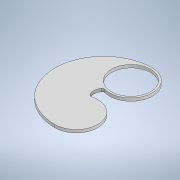
# Autodesk Inventor part: Holder
Saved by Autodesk Inventor 2020 (Build 240168000, 168)
## iProperties
Created: 2020-12-15
Part Number: Holder
Material: Generic
Document SubType Name: Modeling
Designer: moham
Density: 1 g/cm^3
Appearance: Default
Author: moham
Autodesk Inventor part; units mm, degrees
ref_plane "YZ Plane" through (0, 0, 0) normal (1, 0, 0) x (0, 1, 0)
ref_plane "XZ Plane" through (0, 0, 0) normal (0, 1, 0) x (-1, 0, 0)
ref_plane "XY Plane" through (0, 0, 0) normal (0, 0, 1) x (1, 0, 0)
sketch "Sketch1" plane through (0, 0, 0) normal (0, 1, 0) x (-1, 0, 0)
  arc A0 (0, -50) -> (0, 50) centre (0, 0) ccw
  circle A1 centre (0, -28) radius 20
  arc A2 (5.827, -6.7857) -> (0, -50) centre (0, -28) ccw
  arc A3 (0, 50) -> (5.827, 6.7857) centre (0, 28) ccw
  arc A4 (7.9459, -6.0714) -> (7.9459, 6.0714) centre (0, 0) ccw
  arc A5 (7.9459, 6.0714) -> (5.827, 6.7857) centre (6.3567, 4.8571) ccw
  arc A6 (5.827, -6.7857) -> (7.9459, -6.0714) centre (6.3567, -4.8571) ccw
  dimension "d3" = 40
  constraints: 12 point on circle, 7 centre point, 4 tangent, 3 coincident, 1 equal radius
  measures "d3" diameter of A1
extrude "Extrusion1" add sketch "Sketch1" along normal blind 3
body "Solid1"
